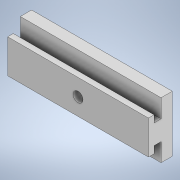
# Autodesk Inventor part: jeep pvc connect on pvc
Saved by Autodesk Inventor 2021 (Build 250183000, 183)
## iProperties
Created: 2020-07-11
Part Number: jeep pvc connect on pvc
Material: Generic
Document SubType Name: Modeling
Designer: Shannon
Density: 1 g/cm^3
Appearance: Default
Author: Shannon
Autodesk Inventor part; units mm, degrees
ref_plane "YZ Plane" through (0, 0, 0) normal (1, 0, 0) x (0, 1, 0)
ref_plane "XZ Plane" through (0, 0, 0) normal (0, 1, 0) x (-1, 0, 0)
ref_plane "XY Plane" through (0, 0, 0) normal (0, 0, 1) x (1, 0, 0)
sketch "Sketch1" plane through (0, 0, 0) normal (0, 0, 1) x (1, 0, 0)
  line L0 (0, 0) -> (127, 0)
  line L1 (127, 0) -> (127, 50.8)
  line L2 (127, 50.8) -> (0, 50.8)
  line L3 (0, 50.8) -> (0, 0)
  dimension "d0" = 50.8
  dimension "d1" = 127
  constraints: 8 end point, 2 parallel, 1 horizontal, 1 perpendicular
  measures "d0" distance between parallel lines of L0 L2
  measures "d1" distance between parallel lines of L1 L3
extrude "Extrusion1" add sketch "Sketch1" along normal blind 10.16
sketch "Sketch2" plane through (0, 0, 10.16) normal (0, 0, 1) x (1, 0, 0)
  line L0 (0, 50.8) -> (0, 0) projected
  line L1 (127, 0) -> (127, 50.8) projected
  line L2 (0, 34.29) -> (127, 34.29)
  line L3 (127, 34.29) -> (127, 16.51)
  line L4 (127, 16.51) -> (0, 16.51)
  line L5 (0, 16.51) -> (0, 34.29)
  line L6 (127, 50.8) -> (0, 50.8) projected
  point P0 (0, 16.51)
  dimension "d4" = 17.78
  dimension "d5" = 16.51
  constraints: 8 end point, 2 parallel, 2 point on line, 1 horizontal, 1 perpendicular
  measures "d4" distance between parallel lines of L4 L2
  measures "d5" distance between parallel lines of L2 L6
extrude "Extrusion2" add sketch "Sketch2" along normal blind 11.43 contours L2 L1 L4 L0
sketch "Sketch4" plane through (0, 34.29, 10.16) normal (0, 1, 0) x (1, 0, 0)
  line L0 (0, 0) -> (0, -11.43) projected
  line L1 (127, 0) -> (127, -11.43) projected
  line L2 (0, -11.43) -> (127, -11.43)
  line L3 (127, -11.43) -> (127, -6.35)
  line L4 (127, -6.35) -> (0, -6.35)
  line L5 (0, -6.35) -> (0, -11.43)
  point P0 (0, 10.16)
  point P1 (0, -6.35)
  dimension "d10" = 5.08
  constraints: 8 end point, 2 parallel, 1 horizontal, 1 perpendicular, 1 point on line
  measures "d10" distance between parallel lines of L4 L2
sketch "Sketch5" plane through (0, 16.51, 10.16) normal (0, -1, 0) x (1, 0, 0)
  line L0 (0, 0) -> (0, 11.43) projected
  line L1 (127, 0) -> (127, 11.43) projected
  line L2 (0, 11.43) -> (127, 11.43)
  line L3 (127, 11.43) -> (127, 6.35)
  line L4 (127, 6.35) -> (0, 6.35)
  line L5 (0, 6.35) -> (0, 11.43)
  point P0 (0, -10.16)
  point P1 (0, 6.35)
  dimension "d11" = 5.08
  constraints: 8 end point, 2 parallel, 1 horizontal, 1 perpendicular, 1 point on line
  measures "d11" distance between parallel lines of L4 L2
extrude "Extrusion3" add sketch "Sketch5" along normal blind 6.35
extrude "Extrusion4" add sketch "Sketch4" along normal blind 6.35
sketch "Sketch6" plane through (0, 0, 0) normal (0, 0, -1) x (-1, 0, 0)
  circle A0 centre (-63.5, 25.4) radius 5.08
  line L0 (0, 50.8) -> (0, 0) projected
  line L1 (0, 0) -> (-127, 0) projected
  dimension "d16" = 10.16
  dimension "d17" = 63.5
  dimension "d18" = 25.4
  constraints: 1 centre point
  measures "d16" diameter of A0
  measures "d17" distance from line of L0 A0.centre
  measures "d18" distance from line of L1 A0.centre
hole "Hole1" at (63.5, 25.4, 0) direction (0, 0, 1) diameter 9.017 end through all
body "Solid1"
